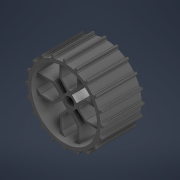
# Autodesk Inventor part: Rover
Saved by Autodesk Inventor 2021 (Build 250183000, 183)
## iProperties
Created: 2020-12-15
Part Number: Rover
Material: Generisch
Document SubType Name: Modeling
Designer: laure
Density: 1 g/cm^3
Appearance: Vorgabe
Author: laure
## iProperties of the stored document _3D-Druck.ipt
Created: 2020-12-29
Part Number: _3D-Druck
Material: Generisch
Document SubType Name: Modeling
Designer: laure
Density: 1 g/cm^3
Appearance: Vorgabe
Author: laure
Autodesk Inventor part; units mm, degrees
ref_plane "YZ Plane" through (0, 0, 0) normal (1, 0, 0) x (0, 1, 0)
ref_plane "XZ Plane" through (0, 0, 0) normal (0, 1, 0) x (-1, 0, 0)
ref_plane "XY Plane" through (0, 0, 0) normal (0, 0, 1) x (1, 0, 0)
sketch "Skizze2" plane through (0, 0, 0) normal (0, 0, 1) x (1, 0, 0)
  circle A0 centre (0, 0) radius 35
  circle A1 centre (0, 0) radius 32
  line L0 (-1.7647, 9.5) -> (-7.5, 16)
  line L1 (-7.5, 28) -> (-7.5, 16)
  line L2 (1.7647, 9.5) -> (7.5, 16)
  line L3 (7.5, 16) -> (7.5, 28)
  line L4 (-9.5, 30.5573) -> (-9.5, 15.2438)
  line L5 (-9.5, 15.2438) -> (-2.3376, 7.1264)
  line L6 (2.3376, 7.1264) -> (9.5, 15.2438)
  line L7 (9.5, 15.2438) -> (9.5, 30.5573)
  circle A2 centre (0, 0) radius 4.5
  line L8 (1.7647, 9.5) -> (-1.7647, 9.5)
  line L9 (-7.1264, -2.3376) -> (-2.3376, -7.1264)
  line L10 (-7.1264, 2.3376) -> (-2.3376, 7.1264)
  line L11 (2.3376, 7.1264) -> (7.1264, 2.3376)
  line L12 (7.1264, -2.3376) -> (2.3376, -7.1264)
  line L13 (-7.5, 28) -> (-4.5, 31.682)
  line L14 (7.5, 28) -> (4.5, 31.682)
  line L15 (-30.5573, -9.5) -> (-15.2438, -9.5)
  line L16 (-28, -7.5) -> (-31.682, -4.5)
  line L17 (-28, -7.5) -> (-16, -7.5)
  line L18 (-9.5, -1.7647) -> (-16, -7.5)
  line L19 (-15.2438, -9.5) -> (-7.1264, -2.3376)
  line L20 (-9.5, 1.7647) -> (-9.5, -1.7647)
  line L21 (-7.1264, 2.3376) -> (-15.2438, 9.5)
  line L22 (-9.5, 1.7647) -> (-16, 7.5)
  line L23 (-15.2438, 9.5) -> (-30.5573, 9.5)
  line L24 (-16, 7.5) -> (-28, 7.5)
  line L25 (-28, 7.5) -> (-31.682, 4.5)
  line L26 (9.5, -30.5573) -> (9.5, -15.2438)
  line L27 (7.5, -28) -> (4.5, -31.682)
  line L28 (7.5, -28) -> (7.5, -16)
  line L29 (1.7647, -9.5) -> (7.5, -16)
  line L30 (9.5, -15.2438) -> (2.3376, -7.1264)
  line L31 (-1.7647, -9.5) -> (1.7647, -9.5)
  line L32 (-2.3376, -7.1264) -> (-9.5, -15.2438)
  line L33 (-1.7647, -9.5) -> (-7.5, -16)
  line L34 (-9.5, -15.2438) -> (-9.5, -30.5573)
  line L35 (-7.5, -16) -> (-7.5, -28)
  line L36 (-7.5, -28) -> (-4.5, -31.682)
  line L37 (30.5573, 9.5) -> (15.2438, 9.5)
  line L38 (28, 7.5) -> (31.682, 4.5)
  line L39 (28, 7.5) -> (16, 7.5)
  line L40 (9.5, 1.7647) -> (16, 7.5)
  line L41 (15.2438, 9.5) -> (7.1264, 2.3376)
  line L42 (9.5, -1.7647) -> (9.5, 1.7647)
  line L43 (7.1264, -2.3376) -> (15.2438, -9.5)
  line L44 (9.5, -1.7647) -> (16, -7.5)
  line L45 (15.2438, -9.5) -> (30.5573, -9.5)
  line L46 (16, -7.5) -> (28, -7.5)
  line L47 (28, -7.5) -> (31.682, -4.5)
  line L48 (-7.1264, 2.3376) -> (-7.1264, -2.3376)
  line L49 (-2.3376, -7.1264) -> (2.3376, -7.1264)
  line L50 (7.1264, -2.3376) -> (7.1264, 2.3376)
  line L51 (2.3376, 7.1264) -> (-2.3376, 7.1264)
  line L52 (0, -49) -> (0, 49) projected
  line L53 (-49, 0) -> (49, 0) projected
  point P0 (-2.3376, -7.1264)
  point P1 (2.3376, -7.1264)
  point P2 (2.3376, -7.1264)
  point P3 (-2.3376, -7.1264)
  dimension "d2" = 70
  dimension "d3" = 3
  dimension "d9" = 2
  dimension "d26" = 360
  dimension "d38" = 9
  constraints: 104 end point, 4 perpendicular, 4 point on circle, 3 centre point, 2 coincident, 2 vertical, 103 other
  measures "d2" diameter of A0
  measures "d3" radial gap between concentric circles of A0 A1
  measures "d9" distance between parallel lines of L1 L4
  measures "d38" diameter of A2
extrude "Extrusion5" add sketch "Skizze2" along normal blind 5 and the other way blind 35 contours L53 A1 L52 A0 | A0 L52 A1 L53 | L52 A1 L53 A0 | A0 L53 A1 L52
extrude "Extrusion7" add sketch "Skizze2" against normal blind 25 contours L38 L39 L40 L42 L53 L50 L41 L37 A1 | A1 L45 L43 L50 L53 L42 L44 L46 L47 | A1 L7 L6 L51 L52 L8 L2 L3 L14 | L13 L1 L0 L8 L52 L51 L5 L4 A1 | A1 L34 L32 L49 L52 L31 L33 L35 L36 | L27 L28 L29 L31 L52 L49 L30 L26 A1 | A1 L23 L21 L48 L53 L20 L22 L24 L25 | L16 L17 L18 L20 L53 L48 L19 L15 A1
extrude "Extrusion8" add sketch "Skizze2" against normal blind 45 contours L53 A2 L52 L51 L11 L50 | L50 L12 L49 L52 A2 L53 | L52 A2 L53 L48 L10 L51 | L49 L9 L48 L53 A2 L52
sketch "Skizze3" plane through (0, 0, -45) normal (0, 0, -1) x (-1, 0, 0)
  circle A0 centre (0, 0) radius 5.2503
  line L0 (2.6105, 0.277) -> (-0.277, -2.6105)
  line L1 (-2.6105, -0.277) -> (0.277, 2.6105)
  arc A1 (-2.6105, -0.277) -> (-0.277, -2.6105) centre (0, 0) ccw
  arc A2 (2.6105, 0.277) -> (0.277, 2.6105) centre (0, 0) ccw
  dimension "d112" = 3.3
  constraints: 4 end point, 4 point on circle, 3 centre point, 2 coincident
  measures "d112" distance between parallel lines of L0 L1
extrude "Extrusion9" add sketch "Skizze3" against normal blind 15
sketch "Skizze9" plane through (0, 0, 5) normal (0, 0, 1) x (1, 0, 0)
  line L0 (-0.5, 37.98) -> (0.5, 37.98)
  line L1 (1, 37.48) -> (1, 34.98)
  line L2 (1, 34.98) -> (-1, 34.98)
  line L3 (-1, 34.98) -> (-1, 37.48)
  line L4 (0, -49.6167) -> (0, 52.7003) projected
  circle A0 centre (0, 0) radius 35 projected
  arc A1 (-0.5, 37.98) -> (-1, 37.48) centre (-0.5, 37.48) ccw
  arc A2 (1, 37.48) -> (0.5, 37.98) centre (0.5, 37.48) ccw
  line L5 (-1, 34.98) -> (-1, 35.98)
  line L6 (-1, 35.98) -> (-1.9442, 34.946)
  line L7 (-1, 34.98) -> (-1.9442, 34.946)
  line L8 (-1, 34.98) -> (-1, 35.98)
  line L9 (1, 34.98) -> (1, 35.98)
  line L10 (1, 35.98) -> (1.9442, 34.946)
  line L11 (1, 34.98) -> (1.9442, 34.946)
  line L12 (1, 34.98) -> (1, 35.98)
  point P0 (1, 37.98)
  point P1 (1, 34.9857)
  point P2 (-1, 34.9857)
  dimension "d102" = 2
  dimension "d103" = 3
  dimension "d104" = 34.98
  dimension "d105" = 0.5
  dimension "d108" = 1
  constraints: 24 end point, 4 point on circle, 4 tangent, 3 point on line, 2 centre point, 2 parallel, 2 symmetric about line, 1 collinear, 1 equal radius, 1 horizontal, 1 perpendicular, 3 other
  measures "d102" distance of L1.end L2.end
  measures "d103" distance of point (1, 37.98) L1.end
  measures "d104" vertical distance of point (0, 0) L2.end
  measures "d105" radius of A1
  measures "d108" distance of L2.end L5.end
extrude "Extrusion11" add sketch "Skizze9" against normal blind 40 contours L0 L4 A0 L3 A1 | L0 A2 L1 A0 L4 | A0 L1 L2 L4 | L4 L2 L3 A0 | L3 A0 L6 | L1 L10 A0
pattern_circular "Runde Anordnung1" count 20 over 360 about axis through (0, 0, 0) along (0, 0, -1) of "Extrusion11"
sketch "Skizze10" plane through (-7.1264, -2.3376, -45) normal (-0.7071, -0.7071, 0) x (0, 0, 1)
  circle A0 centre (5, -3.3865) radius 2
  line L0 (20, 0) -> (0, 0) projected
  line L1 (0, -6.7724) -> (0, 0) projected
  point P0 (45, -3.3862)
  point P1 (45, 0)
  dimension "d113" = 4
  dimension "d114" = 3.3865
  dimension "d115" = 5
  constraints: 1 centre point
  measures "d113" diameter of A0
  measures "d114" distance from line of A0.centre L0
  measures "d115" distance from line of L1 A0.centre
extrude "Extrusion12" cut sketch "Skizze10" against normal up to surface (13.3841 mm away)
